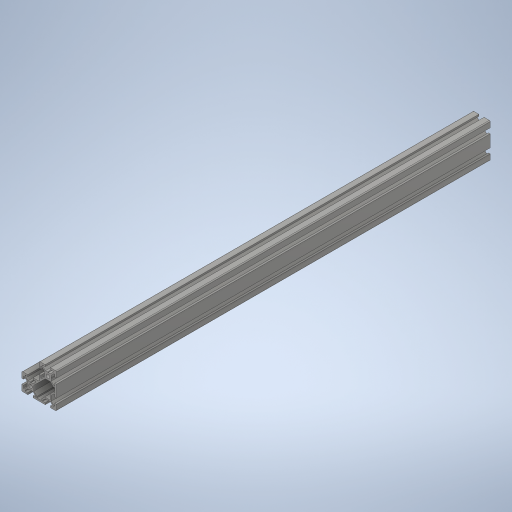
# Autodesk Inventor part: HFS5-404020-500-SC
Saved by Autodesk Inventor 2024 (Build 280153000, 153)
## iProperties
Category: PARTsolutions
Company: MISUMI
Created: 2024-08-01
Part Number: HFS5-404020-500-SC
Material: Aluminum 6061
Catalog Web Link: www.cadenas.de
Description: HFS30A5-20, HFS45A5-20, HFS60A5-20, HFS5-404020, HFSR5-404020, HFSR5-2020-HFS5 Series Aluminum Extrusions 20mm Square -Other Shapes-
Vendor: MISUMI
Document SubType Name: Modeling
Designer: psAdmin
Manufacturer: MISUMI
Mass: 484.75 g
Surface Area: 1827.56 cm^2
Volume: 179.537 cm^3
Density: 2.7 g/cm^3
Appearance: Anodized - Light Gray
PSOL_IDENT_0: {$CADENAS_DATA/23d-libs/misumi/metric/38_al_extrusions_blackets/5/hfs30a5_20.prj},525 {VTYP=3D},{NB=
PSOL_IDENT_1: HFS5-404020-425},{LINA=HFS5-404020-425},{NN=HFS30A5-20, HFS45A5-20, HFS60A5-20, HFS5-404020, HFSR5-4
PSOL_IDENT_2: 04020, HFSR5-2020},{DATE=08.05.2023 08:14:36},{GEOMDATE=27.07.2021 03:20:00},{VERSION=},{LINEID=140}
PSOL_IDENT_3: ,{WBVAR=L,ALT1,ALT2,ALT4,ALT5,CP5,DL5,DR5,ALT6,ALT9,ALT10,ALT11,HP6,NHL6,DL6,NHR6,DR6,ALT7,ALT8,NH9,
PSOL_IDENT_4: AH,BH,CH,DH,EH,NH10,AV,BV,CV,DV,EV,NH11,AP,BP,CP,DP,EP,ALT16,HP16,DL16,DR16,ALT17,HQ17,JLP,ALT18,HQ1
PSOL_IDENT_5: 8,KLP,ALT19,ALT20},{WBNUMERIC=L,NH9,AH,BH,CH,DH,EH,NH10,AV,BV,CV,DV,EV,NH11,AP,BP,CP,DP,EP,HQ17,JLP,
PSOL_IDENT_6: HQ18,KLP}  {NB=HFS5-404020-425},{LINA=HFS5-404020-425},{KT=DUMMY},{PN=HFS5-404020-425},{TPS=HFS5-404
PSOL_IDENT_7: 020},{MAT=A6N01SS-T5 Aluminum Alloy},{ST=Clear Anodize},{FRMW=40},{FRMH=40},{FRD=4.2},{L=425},{MASS=
PSOL_IDENT_8: 1.16},{SA=429},{LX=6.61x10^4},{LY=6.61x10^4},{ALT1=},{M1=0},{DPL1=0},{DPR1=0},{ALT1PN=},{ALT2=},{ALT
PSOL_IDENT_9: 2ALG= '','w/o End Tapping (Heli-Coil Insert)','LHP','with LHP (Tapping on the Left (Heli-Coil Insert
PSOL_IDENT_10: ))','RHP','with RHP (Tapping on the Right (Heli-Coil Insert))','HPW','with HPW (Tapping on Both Ends
PSOL_IDENT_11: (Heli-Coil Insert))' },{M2=0},{DP2=0},{ALT2PN=},{ALT4=},{ALT4ALG= '', 'w/o SC (High Precision Cut)'
PSOL_IDENT_12: , 'SC', 'with SC (High Precision Cut)' },{ALT4PN=},{ALT5=},{ALT5ALG= '','w/o 45 Degree Cut','1','wit
PSOL_IDENT_13: h 45 Degree Cut' },{CP5=},{CP5ALG= '','N/A' },{DL5=},{DL5ALG= '','N/A' },{DR5=},{DR5ALG= '','N/A' },
PSOL_IDENT_14: {FRMLALT5=0},{FRMRALT5=0},{RA5=0},{ALT5PN=},{ALT6=},{ALT6ALG= '','w/o Fastening Location Wrench Acce
PSOL_IDENT_15: ss Hole Alterations','1','with Fastening Location Wrench Access Hole Alterations' },{ALT9=},{ALT9ALG=
PSOL_IDENT_16: '','w/o Location Specified Wrench Access Hole Alteratons (Horizontal)','1','with Location Specified
PSOL_IDENT_17: Wrench Access Hole Alteratons (Horizontal)' },{ALT10=},{ALT10ALG= '','w/o Location Specified Wrench
PSOL_IDENT_18: Access Hole Alteratons (Vertical)','1','with Location Specified Wrench Access Hole Alteratons (Vert
PSOL_IDENT_19: ical)' },{ALT11=},{ALT11ALG= '','w/o Location Specified Wrench Access Hole Alteratons (Crisscross)','
PSOL_IDENT_20: 1','with Location Specified Wrench Access Hole Alteratons (Crisscross)' },{HP6=},{HP6ALG= '','N/A' }
PSOL_IDENT_21: ,{NHL6=},{NHL6ALG= '','N/A' },{DL6=},{DL6ALG= '','N/A' },{NHR6=},{NHR6ALG= '','N/A' },{DR6=},{DR6ALG=
PSOL_IDENT_22: '','N/A' },{HL6=0},{HL6D=0},{HR6=0},{HR6D=0},{J6=0},{J6D=0},{K6=0},{K6D=0},{DD6=0.00},{DD6ALG=0},{A
PSOL_IDENT_23: LT7=},{ALT7ALG= '','N/A' },{ALT8=},{ALT8ALG= '','N/A' },{ALT678PN=},{NH9=0},{NH9MAX=5},{NH9ALG=[0]},
PSOL_IDENT_24: {AH=0.0},{AHMIN=7},{AHMAX=420},{AHALG=[0]},{BH=0.0},{BHMIN=2},{BHMAX=422},{BHALG=[0]},{CH=0.0},{CHMI
PSOL_IDENT_25: N=2},{CHMAX=424},{CHALG=[0]},{DH=0.0},{DHMIN=2},{DHMAX=426},{DHALG=[0]},{EH=0.0},{EHMIN=2},{EHMAX=41
PSOL_IDENT_26: 8},{EHALG=[0]},{NH10=0},{NH10MAX=5},{NH10ALG=[0]},{AV=0.0},{AVMIN=7},{AVMAX=420},{AVALG=[0]},{BV=0.0
PSOL_IDENT_27: },{BVMIN=2},{BVMAX=422},{BVALG=[0]},{CV=0.0},{CVMIN=2},{CVMAX=424},{CVALG=[0]},{DV=0.0},{DVMIN=2},{D
PSOL_IDENT_28: VMAX=426},{DVALG=[0]},{EV=0.0},{EVMIN=2},{EVMAX=418},{EVALG=[0]},{NH11=0},{NH11MAX=5},{NH11ALG=[0]},
PSOL_IDENT_29: {AP=0.0},{APMIN=7},{APMAX=420},{APALG=[0]},{BP=0.0},{BPMIN=2},{BPMAX=422},{BPALG=[0]},{CP=0.0},{CPMI
PSOL_IDENT_30: N=2},{CPMAX=424},{CPALG=[0]},{DP=0.0},{DPMIN=2},{DPMAX=426},{DPALG=[0]},{EP=0.0},{EPMIN=2},{EPMAX=41
PSOL_IDENT_31: 8},{EPALG=[0]},{ALT9PN=},{ALT10PN=},{ALT11PN=},{ALT91011PN=},{ALT16=},{ALT16ALG= '','w/o M Type Hole
PSOL_IDENT_32: Alteration','1','with M Type Hole Alteration' },{HP16=},{HP16ALG= '','N/A' },{DL16=},{DL16ALG= '','
PSOL_IDENT_33: N/A' },{DR16=},{DR16ALG= '','N/A' },{H116=0},{D16=0.0},{ALT16PN=},{ALT17=},{ALT17ALG= '','w/o L Type
PSOL_IDENT_34: Hole Alteration (Top)','1','with L Type Hole Alteration (Top)' },{HQ17=0},{HQ17ALG=0},{JLP=0},{JLPM
PSOL_IDENT_35: IN=4.9},{JLPMAX=0},{JLPALG=[0]},{L17=0},{D17=0.0},{ALT18=},{ALT18ALG= '','w/o L Type Hole Alteration
PSOL_IDENT_36: (Bottom)','1','with L Type Hole Alteration (Bottom)' },{HQ18=0},{HQ18ALG=0},{KLP=0},{KLPMIN=4.9},{K
PSOL_IDENT_37: LPMAX=0},{KLPALG=[0]},{L18=0},{D18=0.0},{ALT1718PN=},{ALT19=},{ALT19ALG= '','N/A' },{M19=0},{DP19=0}
PSOL_IDENT_38: ,{ALT19PN=},{ALT20=},{ALT20PN=},{ERRORALT01=OK},{ERRORALT02=OK},{ERRORALT05=OK},{ERRORALT06091=OK},{
PSOL_IDENT_39: ERRORALT06092=OK},{ERRORALT06093=OK},{ERRORALT06094=OK},{ERRORALT06101=OK},{ERRORALT06102=OK},{ERROR
PSOL_IDENT_40: ALT06103=OK},{ERRORALT06104=OK},{ERRORALT06111=OK},{ERRORALT06112=OK},{ERRORALT06113=OK},{ERRORALT06
PSOL_IDENT_41: 114=OK},{ERRORALT0616=OK},{ERRORALT06171=OK},{ERRORALT06172=OK},{ERRORALT06173=OK},{ERRORALT06181=OK
PSOL_IDENT_42: },{ERRORALT06182=OK},{ERRORALT06183=OK},{ERRORALT0619=OK},{ERRORALT0911=OK},{ERRORALT0916=OK},{ERROR
PSOL_IDENT_43: ALT0917=OK},{ERRORALT0918=OK},{ERRORALT0919=OK},{ERRORALT1011=OK},{ERRORALT1016=OK},{ERRORALT1017=OK
PSOL_IDENT_44: },{ERRORALT1018=OK},{ERRORALT1019=OK},{ERRORALT1116=OK},{ERRORALT1117=OK},{ERRORALT1118=OK},{ERRORAL
PSOL_IDENT_45: T1119=OK},{ERRORALT1617=OK},{ERRORALT1618=OK},{ERRORALT1619=OK},{ERRORALT1719=OK},{ERRORALT1819=OK},
PSOL_IDENT_46: {ERRORPN=},{TFW=0},{IDM1=3.242}
NB: HFS5-404020-425
NN: HFS30A5-20, HFS45A5-20, HFS60A5-20, HFS5-404020, HFSR5-404020, HFSR5-2020
NT: HFS5 Series Aluminum Extrusions 20mm Square -Other Shapes-
NBSYN: $PN.
LINA: HFS5-404020-425
CATALOG: Misumi
PN: HFS5-404020-425
TPS: HFS5-404020
MAT: A6N01SS-T5 Aluminum Alloy
ST: Clear Anodize
L: 425
MASS: 1.16
SA: 429
LX: 6.61x10^4
LY: 6.61x10^4
ALT1: w/o End Tapping
M1: 0
DPL1: 0
DPR1: 0
ALT2: w/o End Tapping (Heli-Coil Insert)
M2: 0
DP2: 0
ALT4: w/o SC (High Precision Cut)
ALT5: w/o 45 Degree Cut
CP5: N/A
DL5: N/A
DR5: N/A
ALT6: w/o Fastening Location Wrench Access Hole Alterations
ALT9: w/o Location Specified Wrench Access Hole Alteratons (Horizontal)
ALT10: w/o Location Specified Wrench Access Hole Alteratons (Vertical)
ALT11: w/o Location Specified Wrench Access Hole Alteratons (Crisscross)
HP6: N/A
NHL6: N/A
DL6: N/A
NHR6: N/A
DR6: N/A
HL6D: 0
HR6D: 0
J6D: 0
K6D: 0
DD6: 0
ALT7: N/A
ALT8: N/A
NH9: 0
AH: 0
BH: 0
CH: 0
DH: 0
EH: 0
NH10: 0
AV: 0
BV: 0
CV: 0
DV: 0
EV: 0
NH11: 0
AP: 0
BP: 0
CP: 0
DP: 0
EP: 0
ALT16: w/o M Type Hole Alteration
HP16: N/A
DL16: N/A
DR16: N/A
H116: 0
D16: 0
ALT17: w/o L Type Hole Alteration (Top)
HQ17: 0
JLP: 0
D17: 0
ALT18: w/o L Type Hole Alteration (Bottom)
HQ18: 0
KLP: 0
D18: 0
ALT19: N/A
M19: 0
ALT20: w/o CW (End Face C Chamfering)
SUPPLIER: MISUMI
ARTICLENO: HFS5-404020-425
BOMINFO: HFS5-404020-425
CREATOR: CADENAS GmbH
Title: HFS5-404020-425
Author: Cadenas PARTsolutions
Comments: HFS5 Series Aluminum Extrusions 20mm Square -Other Shapes-
Autodesk Inventor part; units mm, degrees
ref_plane "YZ Plane" through (0, 0, 0) normal (1, 0, 0) x (0, 1, 0)
ref_plane "XZ Plane" through (0, 0, 0) normal (0, 1, 0) x (-1, 0, 0)
ref_plane "XY Plane" through (0, 0, 0) normal (0, 0, 1) x (1, 0, 0)
sketch "Sketch_1" plane through (0, 0, 0) normal (0, 0, 1) x (1, 0, 0)
  line L0 (-40, 19) -> (-40, 13)
  line L1 (-40, 13) -> (-38, 13)
  line L2 (-38, 13) -> (-38, 16)
  line L3 (-38, 16) -> (-37.0607, 16)
  line L4 (-37.0607, 16) -> (-34, 12.9393)
  line L5 (-34, 12.9393) -> (-34, 10.5196)
  line L6 (-34, 10.5196) -> (-33.7, 10)
  line L7 (-33.7, 10) -> (-34, 9.4804)
  line L8 (-34, 9.4804) -> (-34, 7.0607)
  line L9 (-34, 7.0607) -> (-37.0607, 4)
  line L10 (-37.0607, 4) -> (-38, 4)
  line L11 (-38, 4) -> (-38, 7)
  line L12 (-38, 7) -> (-40, 7)
  line L13 (-40, 7) -> (-40, 1)
  arc A0 (-40, 1) -> (-39, 0) centre (-39, 1) ccw
  line L14 (-39, 0) -> (-33, 0)
  line L15 (-33, 0) -> (-33, 2)
  line L16 (-33, 2) -> (-36, 2)
  line L17 (-36, 2) -> (-36, 2.9393)
  line L18 (-36, 2.9393) -> (-32.9393, 6)
  line L19 (-32.9393, 6) -> (-30.5196, 6)
  line L20 (-30.5196, 6) -> (-30, 6.3)
  line L21 (-30, 6.3) -> (-29.4804, 6)
  line L22 (-29.4804, 6) -> (-27.0607, 6)
  line L23 (-27.0607, 6) -> (-24, 2.9393)
  line L24 (-24, 2.9393) -> (-24, 2)
  line L25 (-24, 2) -> (-27, 2)
  line L26 (-27, 2) -> (-27, 0)
  line L27 (-27, 0) -> (-13, 0)
  line L28 (-13, 0) -> (-13, 2)
  line L29 (-13, 2) -> (-16, 2)
  line L30 (-16, 2) -> (-16, 2.9393)
  line L31 (-16, 2.9393) -> (-12.9393, 6)
  line L32 (-12.9393, 6) -> (-7.0607, 6)
  line L33 (-7.0607, 6) -> (-4, 2.9393)
  line L34 (-4, 2.9393) -> (-4, 2)
  line L35 (-4, 2) -> (-7, 2)
  line L36 (-7, 2) -> (-7, 0)
  line L37 (-7, 0) -> (-1, 0)
  arc A1 (-1, 0) -> (0, 1) centre (-1, 1) ccw
  line L38 (0, 1) -> (0, 7)
  line L39 (0, 7) -> (-2, 7)
  line L40 (-2, 7) -> (-2, 4)
  line L41 (-2, 4) -> (-2.9393, 4)
  line L42 (-2.9393, 4) -> (-6, 7.0607)
  line L43 (-6, 7.0607) -> (-6, 12.9393)
  line L44 (-6, 12.9393) -> (-2.9393, 16)
  line L45 (-2.9393, 16) -> (-2, 16)
  line L46 (-2, 16) -> (-2, 13)
  line L47 (-2, 13) -> (0, 13)
  line L48 (0, 13) -> (0, 27)
  line L49 (0, 27) -> (-2, 27)
  line L50 (-2, 27) -> (-2, 24)
  line L51 (-2, 24) -> (-2.9393, 24)
  line L52 (-2.9393, 24) -> (-6, 27.0607)
  line L53 (-6, 27.0607) -> (-6, 29.4804)
  line L54 (-6, 29.4804) -> (-6.3, 30)
  line L55 (-6.3, 30) -> (-6, 30.5196)
  line L56 (-6, 30.5196) -> (-6, 32.9393)
  line L57 (-6, 32.9393) -> (-2.9393, 36)
  line L58 (-2.9393, 36) -> (-2, 36)
  line L59 (-2, 36) -> (-2, 33)
  line L60 (-2, 33) -> (0, 33)
  line L61 (0, 33) -> (0, 39)
  arc A2 (0, 39) -> (-1, 40) centre (-1, 39) ccw
  line L62 (-1, 40) -> (-7, 40)
  line L63 (-7, 40) -> (-7, 38)
  line L64 (-7, 38) -> (-4, 38)
  line L65 (-4, 38) -> (-4, 37.0607)
  line L66 (-4, 37.0607) -> (-7.0607, 34)
  line L67 (-7.0607, 34) -> (-9.4804, 34)
  line L68 (-9.4804, 34) -> (-10, 33.7)
  line L69 (-10, 33.7) -> (-10.5196, 34)
  line L70 (-10.5196, 34) -> (-12.9393, 34)
  line L71 (-12.9393, 34) -> (-16, 37.0607)
  line L72 (-16, 37.0607) -> (-16, 38)
  line L73 (-16, 38) -> (-13, 38)
  line L74 (-13, 38) -> (-13, 40)
  line L75 (-13, 40) -> (-19, 40)
  arc A3 (-19, 40) -> (-20, 39) centre (-19, 39) ccw
  line L76 (-20, 39) -> (-20, 33)
  line L77 (-20, 33) -> (-18, 33)
  line L78 (-18, 33) -> (-18, 36)
  line L79 (-18, 36) -> (-17.0607, 36)
  line L80 (-17.0607, 36) -> (-14, 32.9393)
  line L81 (-14, 32.9393) -> (-14, 30.5196)
  line L82 (-14, 30.5196) -> (-13.7, 30)
  line L83 (-13.7, 30) -> (-14, 29.4804)
  line L84 (-14, 29.4804) -> (-14, 27.0607)
  line L85 (-14, 27.0607) -> (-17.0607, 24)
  line L86 (-17.0607, 24) -> (-18, 24)
  line L87 (-18, 24) -> (-18, 27)
  line L88 (-18, 27) -> (-20, 27)
  line L89 (-20, 27) -> (-20, 20.3)
  arc A4 (-20.3, 20) -> (-20, 20.3) centre (-20.3, 20.3) ccw
  line L90 (-20.3, 20) -> (-27, 20)
  line L91 (-27, 20) -> (-27, 18)
  line L92 (-27, 18) -> (-24, 18)
  line L93 (-24, 18) -> (-24, 17.0607)
  line L94 (-24, 17.0607) -> (-27.0607, 14)
  line L95 (-27.0607, 14) -> (-29.4804, 14)
  line L96 (-29.4804, 14) -> (-30, 13.7)
  line L97 (-30, 13.7) -> (-30.5196, 14)
  line L98 (-30.5196, 14) -> (-32.9393, 14)
  line L99 (-32.9393, 14) -> (-36, 17.0607)
  line L100 (-36, 17.0607) -> (-36, 18)
  line L101 (-36, 18) -> (-33, 18)
  line L102 (-33, 18) -> (-33, 20)
  line L103 (-33, 20) -> (-39, 20)
  arc A5 (-39, 20) -> (-40, 19) centre (-39, 19) ccw
  line L104 (-26, 7.0607) -> (-22.5, 3.5607)
  line L105 (-22.5, 3.5607) -> (-22.5, 2)
  line L106 (-22.5, 2) -> (-17.5, 2)
  line L107 (-17.5, 2) -> (-17.5, 3.5607)
  line L108 (-17.5, 3.5607) -> (-13.5607, 7.5)
  line L109 (-13.5607, 7.5) -> (-7.5, 7.5)
  line L110 (-7.5, 7.5) -> (-7.5, 13.5607)
  line L111 (-7.5, 13.5607) -> (-3.5607, 17.5)
  line L112 (-3.5607, 17.5) -> (-2, 17.5)
  line L113 (-2, 17.5) -> (-2, 22.5)
  line L114 (-2, 22.5) -> (-3.5607, 22.5)
  line L115 (-3.5607, 22.5) -> (-7.0607, 26)
  line L116 (-7.0607, 26) -> (-12.9393, 26)
  line L117 (-12.9393, 26) -> (-26, 12.9393)
  line L118 (-26, 12.9393) -> (-26, 7.0607)
  constraints: 238 end point, 12 point on circle, 6 centre point
extrude "Extrusion1" add sketch "Sketch_1" against normal blind 500
sketch "Sketch2" plane through (0, 0, -500) normal (0, 0, -1) x (-1, 0, 0)
  point P0 (10, 30)
hole "Hole1" at (-10, 30, -500) direction (0, 0, 1) diameter 4.2 end through all
sketch "Sketch3" plane through (0, 0, -500) normal (0, 0, -1) x (-1, 0, 0)
  point P0 (30, 10)
hole "Hole2" at (-30, 10, -500) direction (0, 0, 1) diameter 4.2 end through all
thread "Thread1" size "M5x0.8" class "6H" standard "ANSI Metric M Profile" length 10
thread "Thread2" size "M5x0.8" class "6H" standard "ANSI Metric M Profile" length 10
thread "Thread3" size "M5x0.8" class "6H" standard "ANSI Metric M Profile" length 10
thread "Thread4" size "M5x0.8" class "6H" standard "ANSI Metric M Profile" length 10
body "Solid1"
